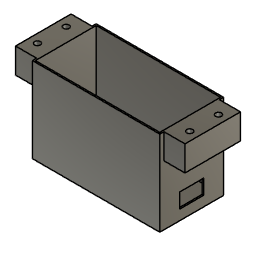
Large Servo Box v3 (Autodesk Fusion 360 design; units mm, degrees)
Autodesk Fusion 360 part; units mm, degrees
sketch "Sketch1" plane through (0, 0, 0) normal (0, 0, 1) x (1, 0, 0)
  line L0 (-25, -19.2) -> (-25, 2.3)
  line L1 (-25, 2.3) -> (17.94, 2.3)
  line L2 (17.94, 2.3) -> (17.94, -19.2)
  line L3 (17.94, -19.2) -> (-25, -19.2)
  dimension "d1" = 21.5
  dimension "d2" = 42.94
  constraint perpendicular L0 L1
  constraint perpendicular L1 L2
  constraint perpendicular L0 L3
  measures "d1" distance of L0.start L0.end
  measures "d2" distance of L0.end L1.end
extrude "Extrude1" add sketch "Sketch1" along normal blind 28.65
shell "Shell1" thickness 0.5 removed faces 1 at (3.6267, -12.0333, 28.65)
sketch "Sketch2" plane through (17.94, 0, 0) normal (1, 0, 0) x (0, 1, 0)
  line L0 (-19.2, 0) -> (2.3, 0)
  line L1 (2.3, 0) -> (2.3, 28.65)
  line L2 (2.3, 28.65) -> (-19.2, 28.65)
  line L3 (-19.2, 28.65) -> (-19.2, 0)
  line L4 (-12.5, 8.4) -> (-4.4, 8.4)
  line L5 (-4.4, 8.4) -> (-4.4, 3.4)
  line L6 (-4.4, 3.4) -> (-12.5, 3.4)
  line L7 (-12.5, 3.4) -> (-12.5, 8.4)
  dimension "d6" = 3.4
  dimension "d7" = 8.1
  dimension "d8" = 6.7
  dimension "d9" = 6.7
  dimension "d39" = 5
  constraint horizontal L4
  constraint vertical L5
  constraint horizontal L6
  constraint vertical L7
  measures "d6" distance of L0 L6
  measures "d7" distance of L4.start L4.end
  measures "d8" distance of L3 L7
  measures "d9" distance of L1 L5
  measures "d39" distance of L4.start L6.end
extrude "Extrude2" cut sketch "Sketch2" along normal mid plane 6 contours L4 L5 L6 L7
sketch "Sketch3" plane through (17.94, 0, 0) normal (1, 0, 0) x (0, 1, 0)
  line L0 (-4.4, 8.4) -> (-4.4, 3.4)
  line L1 (-4.4, 3.4) -> (-12.5, 3.4)
  line L2 (-12.5, 3.4) -> (-12.5, 8.4)
  line L3 (-12.5, 8.4) -> (-4.4, 8.4)
  line L4 (-19.2, 0) -> (2.3, 0)
  line L5 (2.3, 0) -> (2.3, 28.65)
  line L6 (2.3, 28.65) -> (-19.2, 28.65)
  line L7 (-19.2, 28.65) -> (-19.2, 0)
  line L8 (-17.8, 28.65) -> (0.9, 28.65)
  line L9 (0.9, 28.65) -> (0.9, 20.15)
  line L10 (0.9, 20.15) -> (-17.8, 20.15)
  line L11 (-17.8, 20.15) -> (-17.8, 28.65)
  dimension "d19" = 18.7
  dimension "d20" = 1.4
  dimension "d23" = 8.5
  constraint horizontal L8
  constraint vertical L9
  constraint horizontal L10
  constraint vertical L11
  constraint coincident L6 L8.start
  measures "d19" distance of L9.end L10.end
  measures "d20" distance of L5 L9
  measures "d23" distance of L8.start L10.end
extrude "Extrude3" add sketch "Sketch3" along normal blind 7.1 contours L6 L8 L9 L10 L11
sketch "Sketch4" plane through (0, 0, 28.65) normal (0, 0, 1) x (-1, 0, 0)
  line L0 (-17.44, 18.7) -> (24.5, 18.7)
  line L1 (24.5, 18.7) -> (24.5, -1.8)
  line L2 (24.5, -1.8) -> (-17.44, -1.8)
  line L3 (-17.44, -1.8) -> (-17.44, 18.7)
  line L4 (-17.94, 19.2) -> (-17.94, 17.8)
  line L5 (-17.94, 17.8) -> (-25.04, 17.8)
  line L6 (-25.04, 17.8) -> (-25.04, -0.9)
  line L7 (-25.04, -0.9) -> (-17.94, -0.9)
  line L8 (-17.94, -0.9) -> (-17.94, -2.3)
  line L9 (-17.94, -2.3) -> (25, -2.3)
  line L10 (25, -2.3) -> (25, 19.2)
  line L11 (25, 19.2) -> (-17.94, 19.2)
  circle A0 centre (-22.15, 3.6) radius 2.25
  circle A1 centre (-22.15, 13.3) radius 2.25
  dimension "d40" = 4.5
  dimension "d41" = 4.5
  dimension "d44" = 9.7
  dimension "d45" = 4.71
  dimension "d46" = 4.71
  dimension "d47" = 4.5
  measures "d40" diameter of A1
  measures "d41" diameter of A0
  measures "d44" distance of A0.centre A1.centre
  measures "d45" distance of L3 A0.centre
  measures "d46" distance of L3 A1.centre
  measures "d47" distance of L7 A0.centre
sketch "Sketch6" plane through (-25, 0, 0) normal (-1, 0, 0) x (0, -1, 0)
  line L0 (-2.3, 0) -> (19.2, 0)
  line L1 (19.2, 0) -> (19.2, 28.65)
  line L2 (19.2, 28.65) -> (-2.3, 28.65)
  line L3 (-2.3, 28.65) -> (-2.3, 0)
  line L4 (-0.9, 28.65) -> (17.8, 28.65)
  line L5 (17.8, 28.65) -> (17.8, 20.15)
  line L6 (17.8, 20.15) -> (-0.9, 20.15)
  line L7 (-0.9, 20.15) -> (-0.9, 28.65)
  dimension "d27" = 1.4
  dimension "d28" = 18.7
  dimension "d29" = 8.5
  constraint horizontal L4
  constraint vertical L5
  constraint horizontal L6
  constraint vertical L7
  constraint coincident L2 L4.start
  measures "d27" distance of L1 L5
  measures "d28" distance of L5.end L6.end
  measures "d29" distance of L4.start L6.end
extrude "Extrude5" add sketch "Sketch6" along normal blind 7.1 contours L2 L4 L5 L6 L7
sketch "Sketch7" plane through (0, 0, 28.65) normal (0, 0, 1) x (-1, 0, 0)
  line L0 (-17.44, 18.7) -> (24.5, 18.7)
  line L1 (24.5, 18.7) -> (24.5, -1.8)
  line L2 (24.5, -1.8) -> (-17.44, -1.8)
  line L3 (-17.44, -1.8) -> (-17.44, 18.7)
  line L4 (-17.94, 19.2) -> (-17.94, 17.8)
  line L5 (-17.94, 17.8) -> (-25.04, 17.8)
  line L6 (-25.04, 17.8) -> (-25.04, -0.9)
  line L7 (-25.04, -0.9) -> (-17.94, -0.9)
  line L8 (-17.94, -0.9) -> (-17.94, -2.3)
  line L9 (-17.94, -2.3) -> (25, -2.3)
  line L10 (25, -2.3) -> (25, -0.9)
  line L11 (25, -0.9) -> (32.1, -0.9)
  line L12 (32.1, -0.9) -> (32.1, 17.8)
  line L13 (32.1, 17.8) -> (25, 17.8)
  line L14 (25, 17.8) -> (25, 19.2)
  line L15 (25, 19.2) -> (-17.94, 19.2)
  circle A0 centre (26.6, 4.1) radius 1.025
  dimension "d34" = 2.05
  dimension "d35" = 2.1
  dimension "d36" = 5
  measures "d34" diameter of A0
  measures "d35" distance of L1 A0.centre
  measures "d36" distance of L11 A0.centre
sketch "Sketch8" plane through (0, 0, 28.65) normal (0, 0, 1) x (-1, 0, 0)
  line L0 (-17.44, 18.7) -> (24.5, 18.7)
  line L1 (24.5, 18.7) -> (24.5, -1.8)
  line L2 (24.5, -1.8) -> (-17.44, -1.8)
  line L3 (-17.44, -1.8) -> (-17.44, 18.7)
  line L4 (-17.94, 19.2) -> (-17.94, 17.8)
  line L5 (-17.94, 17.8) -> (-25.04, 17.8)
  line L6 (-25.04, 17.8) -> (-25.04, -0.9)
  line L7 (-25.04, -0.9) -> (-17.94, -0.9)
  line L8 (-17.94, -0.9) -> (-17.94, -2.3)
  line L9 (-17.94, -2.3) -> (25, -2.3)
  line L10 (25, -2.3) -> (25, -0.9)
  line L11 (25, -0.9) -> (32.1, -0.9)
  line L12 (32.1, -0.9) -> (32.1, 17.8)
  line L13 (32.1, 17.8) -> (25, 17.8)
  line L14 (25, 17.8) -> (25, 19.2)
  line L15 (25, 19.2) -> (-17.94, 19.2)
  circle A0 centre (-22.15, 3.6) radius 1
  circle A1 centre (-22.15, 13.3) radius 1
  circle A2 centre (29.21, 3.6) radius 1
  circle A3 centre (29.21, 13.3) radius 1
  dimension "d48" = 2
  dimension "d49" = 2
  dimension "d50" = 4.71
  dimension "d51" = 9.7
  dimension "d52" = 4.5
  dimension "d53" = 4.71
  dimension "d54" = 2
  dimension "d55" = 2
  dimension "d56" = 9.7
  dimension "d57" = 4.71
  dimension "d58" = 4.5
  dimension "d59" = 4.71
  measures "d48" diameter of A0
  measures "d49" diameter of A1
  measures "d50" distance of L3 A0.centre
  measures "d51" vertical distance of A0.centre A1.centre
  measures "d52" distance of L5 A1.centre
  measures "d53" distance of L3 A1.centre
  measures "d54" diameter of A2
  measures "d55" diameter of A3
  measures "d56" distance of A2.centre A3.centre
  measures "d57" distance of L1 A3.centre
  measures "d58" distance of L13 A3.centre
  measures "d59" distance of L1 A2.centre
extrude "Extrude7" cut sketch "Sketch8" against normal blind 8.65 contours A0 | A1 | A2 | A3
